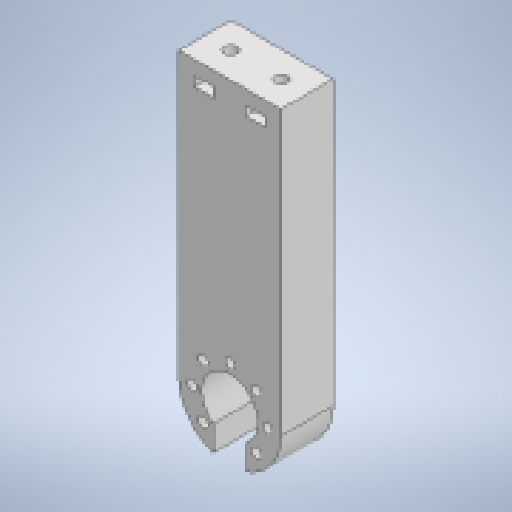
# Autodesk Inventor part: _hand_1_
Saved by Autodesk Inventor 2024.3 (Build 283343000, 343)
## iProperties
Created: 2024-09-06
Part Number: _hand_1_
Material: 일반
Document SubType Name: Modeling
Designer: gretc
Density: 1 g/cm^3
Appearance: 기본값
Mass: 14.269 g
Surface Area: 57.0929 cm^2
Volume: 14.269 cm^3
Author: gretc
Autodesk Inventor part; units mm, degrees
ref_plane "YZ Plane" through (0, 0, 0) normal (1, 0, 0) x (0, 1, 0)
ref_plane "XZ Plane" through (0, 0, 0) normal (0, 1, 0) x (-1, 0, 0)
ref_plane "XY Plane" through (0, 0, 0) normal (0, 0, 1) x (1, 0, 0)
sketch "스케치1" plane through (0, 0, 0) normal (0, 0, 1) x (1, 0, 0)
  circle A0 centre (0, 0) radius 10.8 projected
  circle A1 centre (0, 0) radius 6 projected
  circle A2 centre (0, -8) radius 1.05 projected
  circle A3 centre (-5.6569, -5.6569) radius 1.05 projected
  circle A4 centre (-8, 0) radius 1.05 projected
  circle A5 centre (-5.6569, 5.6569) radius 1.05 projected
  circle A6 centre (0, 8) radius 1.05 projected
  circle A7 centre (5.6569, 5.6569) radius 1.05 projected
  circle A8 centre (8, 0) radius 1.05 projected
  circle A9 centre (5.6569, -5.6569) radius 1.05 projected
  circle A10 centre (0, 0) radius 3 projected
  circle A11 centre (0, 0) radius 3.5 projected
  line L0 (3.5, 0) -> (-3.5, 0)
  line L1 (-3.5, 0) -> (-3.5, -11.2226)
  line L2 (-3.5, -11.2226) -> (3.5, -11.2226)
  line L3 (3.5, -11.2226) -> (3.5, 0)
  line L4 (10.8, 0) -> (-10.8, 0)
  line L5 (-10.8, 0) -> (-10.8, 60)
  line L6 (-10.8, 60) -> (10.8, 60)
  line L7 (10.8, 60) -> (10.8, 0)
  point P0 (0, 0)
  point P1 (3.5, -4.8734)
  point P2 (3.5, -10.2171)
  point P3 (-3.5, -10.2171)
  point P4 (-3.5, -4.8734)
  dimension "d0" = 60
  constraints: 16 end point, 4 parallel, 4 point on circle, 2 perpendicular, 1 horizontal, 1 point on line
  measures "d0" distance of L4.end L5.end
extrude "돌출1" add sketch "스케치1" along normal blind 11.0652 contours L4 A8 A1 A4 A0 | A0 L3 A1 L4 A8 | A0 L5 L6 L7 | L4 A4 A1 L1 A0
sketch "스케치2" plane through (-10.8, 60, 0) normal (0, 1, 0) x (1, 0, 0)
  circle A0 centre (16.2, -5.5326) radius 1.35 projected
  circle A1 centre (5.4, -5.5326) radius 1.35 projected
  point P0 (10.8, 0)
extrude "돌출2" cut sketch "스케치2" against normal blind 4
sketch "스케치3" plane through (0, 0, 11.0652) normal (0, 0, 1) x (1, 0, 0)
  line L0 (4.05, 56) -> (6.75, 56) projected
  line L1 (-6.75, 56) -> (-4.05, 56) projected
  line L2 (-6.75, 60) -> (-6.75, 56) projected
  line L3 (-4.05, 60) -> (-4.05, 56) projected
  line L4 (4.05, 60) -> (4.05, 56) projected
  line L5 (6.75, 60) -> (6.75, 56) projected
  line L6 (3.4, 55) -> (7.4, 55)
  line L7 (7.4, 55) -> (7.4, 57)
  line L8 (7.4, 57) -> (3.4, 57)
  line L9 (3.4, 57) -> (3.4, 55)
  line L10 (3.4, 55) -> (7.4, 57) construction
  line L11 (7.4, 55) -> (3.4, 57) construction
  line L12 (-7.4, 55) -> (-3.4, 55)
  line L13 (-3.4, 55) -> (-3.4, 57)
  line L14 (-3.4, 57) -> (-7.4, 57)
  line L15 (-7.4, 57) -> (-7.4, 55)
  line L16 (-7.4, 55) -> (-3.4, 57) construction
  line L17 (-3.4, 55) -> (-7.4, 57) construction
  point P0 (0, 0)
  point P1 (5.4, 56)
  point P2 (-5.4, 56)
  dimension "d5" = 4
  dimension "d6" = 2
  dimension "d7" = 4
  dimension "d8" = 2
  constraints: 24 end point, 6 midpoint, 4 parallel, 2 perpendicular
  measures "d5" distance of L6.start L6.end
  measures "d6" distance of L7.end L6.end
  measures "d7" distance of L12.start L12.end
  measures "d8" distance of L13.end L12.end
extrude "돌출3" cut sketch "스케치3" against normal blind 10
